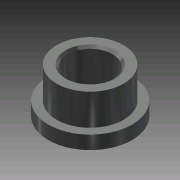
# Autodesk Inventor part: Ratchet Bushing 1764
Saved by Autodesk Inventor 2011 (Build 150239000, 239)
## iProperties
Created: 2010-02-05
Part Number: Ratchet Bushing 1764
Document SubType Name: Modeling
Designer: jrobinson
Density: 1 g/cm^3
Author: jrobinson
Autodesk Inventor part; units mm, degrees
ref_plane "YZ Plane" through (0, 0, 0) normal (1, 0, 0) x (0, 1, 0)
ref_plane "XZ Plane" through (0, 0, 0) normal (0, 1, 0) x (-1, 0, 0)
ref_plane "XY Plane" through (0, 0, 0) normal (0, 0, 1) x (1, 0, 0)
sketch "Sketch1" plane through (0, 0, 0) normal (0, 0, 1) x (1, 0, 0)
  line L0 (-4.6769, 8.9222) -> (-7.8519, 8.9222)
  line L1 (-7.8519, 8.9222) -> (-7.8519, 0.0322)
  line L2 (-7.8519, -3.7778) -> (-4.6769, -3.7778)
  line L3 (1.6731, -3.7778) -> (1.6731, 8.9222)
  line L4 (-4.6769, -3.7778) -> (-10.2395, -3.7778)
  line L5 (-10.2395, -3.7778) -> (-10.2395, 0.0322)
  line L6 (-10.2395, 0.0322) -> (-7.8519, 0.0322)
  line L7 (1.6731, 3.6296) -> (1.6731, -3.7778)
  line L8 (-4.6769, -3.7778) -> (-4.6769, 8.9222)
  point P0 (0, 0)
  dimension "d0" = 12.7
  dimension "d1" = 11.9126
  dimension "d2" = 9.525
  dimension "d3" = 6.35
  dimension "d4" = 3.81
  constraints: 18 end point, 4 parallel, 3 perpendicular, 2 horizontal
  measures "d0" distance between parallel lines of L4 L0
  measures "d1" distance of L3.start L4.end
  measures "d2" distance between parallel lines of L3 L1
  measures "d3" distance between parallel lines of L3 L8
  measures "d4" distance of L4.end L5.end
revolve "Revolution1" add sketch "Sketch1" angle 360 about axis through (1.6731, -3.7778, 0) along (0, 1, 0)
chamfer "Chamfer1" distance 0.635 angle 45 1 edges at (8.0231, 8.9222, 0)
fillet "Fillet1" radius 0.127 1 edges at (8.0231, -3.7778, 0)
body "Solid1"
